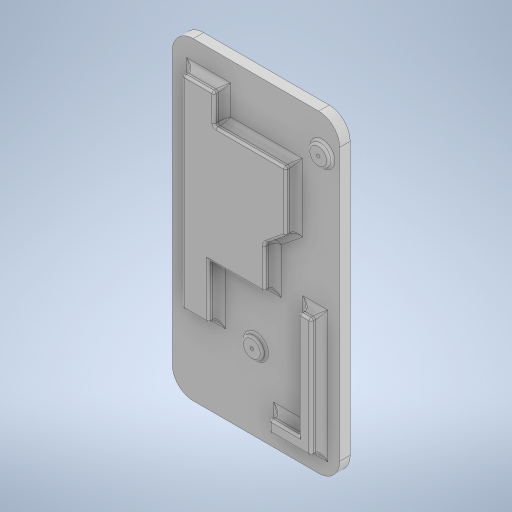
# Autodesk Inventor part: aluminium_plate
Saved by Autodesk Inventor 2024.3 (Build 283343000, 343)
## iProperties
Created: 2025-09-03
Part Number: aluminium_plate
Material: Generico
Document SubType Name: Modeling
Designer: chris
Density: 1 g/cm^3
Appearance: Default
Author: chris
Autodesk Inventor part; units mm, degrees
ref_plane "YZ Plane" through (0, 0, 0) normal (1, 0, 0) x (0, 1, 0)
ref_plane "XZ Plane" through (0, 0, 0) normal (0, 1, 0) x (-1, 0, 0)
ref_plane "XY Plane" through (0, 0, 0) normal (0, 0, 1) x (1, 0, 0)
sketch "Schizzo1" plane through (0, 0, 0) normal (0, 0, 1) x (1, 0, 0)
  line L0 (0.4, 0.75) -> (-0.4, 0.75)
  line L1 (-0.4, 0.75) -> (-0.4, -0.75)
  line L2 (-0.4, -0.75) -> (0.4, -0.75)
  line L3 (0.4, -0.75) -> (0.4, 0.75)
  line L4 (0.4, 0.75) -> (-0.4, -0.75) construction
  line L5 (-0.4, 0.75) -> (0.4, -0.75) construction
  point P0 (0, 0)
  dimension "d0" = 1.5
  dimension "d1" = 0.8
  constraints: 12 end point, 2 midpoint, 2 parallel, 1 horizontal, 1 perpendicular
  measures "d0" distance of L0.end L1.end
  measures "d1" distance of L1.end L2.end
extrude "Estrusione1" add sketch "Schizzo1" along normal blind 0.05
sketch "Schizzo2" plane through (0, 0, 0.05) normal (0, 0, 1) x (1, 0, 0)
  line L0 (-0.4, 0.75) -> (-0.4, -0.75) construction
  line L1 (-0.4, -0.75) -> (0.4, -0.75) construction
  line L2 (0.4, -0.75) -> (0.4, 0.75) construction
  line L3 (0.4, 0.75) -> (-0.4, 0.75) construction
  line L4 (-0.3016, -0.3447) -> (-0.1759, -0.3447)
  line L5 (-0.1759, -0.3447) -> (-0.1759, -0.082)
  line L6 (-0.1759, -0.082) -> (0.0902, -0.082)
  line L7 (0.0902, -0.082) -> (0.0902, 0.1207)
  line L8 (0.0902, 0.1207) -> (0.1921, 0.2033)
  line L9 (0.1921, 0.2033) -> (0.1921, 0.4853)
  line L10 (0.1921, 0.4853) -> (-0.151, 0.4853)
  line L11 (-0.151, 0.4853) -> (-0.151, 0.6264)
  line L12 (-0.151, 0.6264) -> (-0.3016, 0.6264)
  line L13 (-0.3016, 0.6264) -> (-0.3016, -0.3447)
  line L14 (0.114, -0.6516) -> (0.3133, -0.6516)
  line L15 (0.3133, -0.6516) -> (0.3133, -0.082)
  line L16 (0.3133, -0.082) -> (0.2546, -0.082)
  line L17 (0.2546, -0.082) -> (0.2546, -0.5927)
  line L18 (0.2546, -0.5927) -> (0.114, -0.5927)
  line L19 (0.114, -0.6516) -> (0.114, -0.5927)
  point P0 (0, 0)
  constraints: 32 end point, 11 perpendicular, 2 horizontal, 1 parallel, 1 vertical
extrude "Estrusione2" add sketch "Schizzo2" along normal blind 0.05
fillet "Raccordo1" radius 0.03 3 edges at (0.0902, 0.0193, 0.05) (-0.1759, -0.2134, 0.05) (-0.0429, -0.082, 0.05)
fillet "Raccordo2" radius 0.03 15 edges at (0.099, 0.1278, 0.0588) (0.0902, 0.1207, 0.09) (0.1562, 0.1742, 0.05) (0.1921, 0.3443, 0.05) (0.0206, 0.4853, 0.05) (-0.151, 0.5558, 0.05) (-0.2263, 0.6264, 0.05) (-0.3016, 0.1408, 0.05) (-0.2388, -0.3447, 0.05) (0.2136, -0.6516, 0.05) (0.3133, -0.3668, 0.05) (0.2839, -0.082, 0.05) (0.2546, -0.3374, 0.05) (0.1843, -0.5927, 0.05) (0.114, -0.6222, 0.05)
fillet "Raccordo3" radius 0.01 14 edges at (0.3221, -0.0732, 0.0588) (0.3133, -0.082, 0.09) (0.2458, -0.0732, 0.0588) (0.2546, -0.082, 0.09) (0.3221, -0.6604, 0.0588) (0.3133, -0.6516, 0.09) (0.1052, -0.6604, 0.0588) (0.114, -0.6516, 0.09) (0.1052, -0.5839, 0.0588) (0.114, -0.5927, 0.09) (0.3133, -0.3668, 0.1) (0.2546, -0.3374, 0.1) (0.1843, -0.5927, 0.1) (0.2136, -0.6516, 0.1)
fillet "Raccordo4" radius 0.01 6 edges at (0.1169, -0.6487, 0.0971) (0.1169, -0.5957, 0.0971) (0.114, -0.6222, 0.1) (0.2575, -0.0849, 0.0971) (0.3104, -0.0849, 0.0971) (0.2839, -0.082, 0.1)
fillet "Raccordo5" radius 0.01 27 edges at (0.0931, 0.1193, 0.1) (0.1467, 0.1665, 0.1) (0.0902, 0.0122, 0.1) (0.1921, 0.3443, 0.1) (0.0206, 0.4853, 0.1) (-0.151, 0.5558, 0.1) (-0.2263, 0.6264, 0.1) (-0.3016, 0.1408, 0.1) (-0.2388, -0.3447, 0.1) (-0.1759, -0.2134, 0.1) (-0.0429, -0.082, 0.1) (0.2009, 0.4941, 0.0588) (0.1921, 0.4853, 0.09) (-0.1422, 0.4941, 0.0588) (-0.151, 0.4853, 0.09) (-0.1422, 0.6352, 0.0588) (-0.151, 0.6264, 0.09) (-0.3104, 0.6352, 0.0588) (-0.3016, 0.6264, 0.09) (0.2009, 0.1992, 0.0588) (0.1921, 0.2033, 0.09) (0.099, -0.0908, 0.0588) (0.0902, -0.082, 0.09) (-0.1759, -0.3447, 0.09) (-0.1671, -0.3535, 0.0588) (-0.3104, -0.3535, 0.0588) (-0.3016, -0.3447, 0.09)
sketch "Schizzo3" plane through (0, 0, 0.05) normal (0, 0, 1) x (1, 0, 0)
  circle A0 centre (0, -0.3735) radius 0.05
  circle A1 centre (0.3174, 0.5827) radius 0.05
  point P0 (0, 0)
  dimension "d11" = 0.1
  dimension "d12" = 0.1
  constraints: 2 centre point
  measures "d11" diameter of A0
  measures "d12" diameter of A1
extrude "Estrusione3" add sketch "Schizzo3" along normal blind 0.02
fillet "Raccordo6" radius 0.01 2 edges at (0.2674, 0.5827, 0.05) (-0.05, -0.3735, 0.05)
sketch "Schizzo4" plane through (0, -0.3735, 0.07) normal (0, 0, 1) x (1, 0, 0)
  circle A0 centre (0, 0) radius 0.0075
  circle A1 centre (0.3174, 0.9562) radius 0.05 construction
  circle A2 centre (0, 0) radius 0.05 construction
  circle A3 centre (0.3174, 0.9562) radius 0.0075
  point P0 (0, 0.3735)
  dimension "d16" = 0.015
  dimension "d17" = 0.015
  constraints: 2 centre point, 1 coincident
  measures "d16" diameter of A0
  measures "d17" diameter of A3
extrude "Estrusione4" cut sketch "Schizzo4" against normal through all
fillet "Raccordo7" radius 0.01 2 edges at (-0.05, -0.3735, 0.07) (0.2674, 0.5827, 0.07)
fillet "Raccordo8" radius 0.1 4 edges at (0.4, 0.75, 0.025) (-0.4, 0.75, 0.025) (-0.4, -0.75, 0.025) (0.4, -0.75, 0.025)
